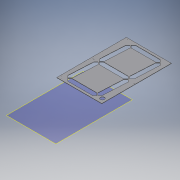
# Autodesk Inventor part: Cover_V2
Saved by Autodesk Inventor 2016 SP2 (Build 200236200, 236)
## iProperties
Created: 2018-06-10
Part Number: Cover_V2
Material: Generisch
Document SubType Name: Modeling
Designer: Nils
Density: 1 g/cm^3
Appearance: Vorgabe
Author: Nils
Autodesk Inventor part; units mm, degrees
ref_plane "YZ Plane" through (0, 0, 0) normal (1, 0, 0) x (0, 1, 0)
ref_plane "XZ Plane" through (0, 0, 0) normal (0, 1, 0) x (-1, 0, 0)
ref_plane "XY Plane" through (0, 0, 0) normal (0, 0, 1) x (1, 0, 0)
sketch "Skizze1" plane through (0, 0, 0) normal (0, 0, 1) x (1, 0, 0)
  line L0 (-29.0874, 239.038) -> (-29.0874, 85.837) projected
  line L1 (-29.0874, 85.837) -> (69.9128, 85.837) projected
  line L2 (-21.0874, 102.0037) -> (-18.2612, 155.9297) projected
  line L3 (-16.0874, 97.0037) -> (-21.0874, 102.0037) projected
  line L4 (-11.0874, 102.0037) -> (-16.0874, 97.0037) projected
  line L5 (-18.2612, 155.9297) -> (-13.2612, 160.9297) projected
  line L6 (-13.2612, 160.9297) -> (-8.2612, 155.9297) projected
  line L7 (44.0794, 90.837) -> (-9.9206, 90.837) projected
  line L8 (-9.9206, 90.837) -> (-14.9206, 95.837) projected
  line L9 (-14.9206, 95.837) -> (-9.9206, 100.837) projected
  line L10 (49.0794, 95.837) -> (44.0794, 90.837) projected
  line L11 (44.0794, 100.837) -> (49.0794, 95.837) projected
  line L12 (-9.9206, 100.837) -> (44.0794, 100.837)
  line L13 (-11.0874, 102.0037) -> (-8.2612, 155.9297)
  line L14 (-17.5791, 168.9453) -> (-14.753, 222.8713) projected
  line L15 (-12.5791, 163.9453) -> (-17.5791, 168.9453) projected
  line L16 (-7.5791, 168.9453) -> (-12.5791, 163.9453) projected
  line L17 (-14.753, 222.8713) -> (-9.753, 227.8713) projected
  line L18 (-9.753, 227.8713) -> (-4.753, 222.8713) projected
  line L19 (-3.5862, 224.038) -> (-8.5862, 229.038) projected
  line L20 (-8.5862, 229.038) -> (-3.5862, 234.038) projected
  line L21 (-3.5862, 234.038) -> (50.4138, 234.038) projected
  line L22 (50.4138, 234.038) -> (55.4138, 229.038) projected
  line L23 (55.4138, 229.038) -> (50.4138, 224.038) projected
  line L24 (51.5805, 222.8713) -> (56.5805, 227.8713) projected
  line L25 (56.5805, 227.8713) -> (61.5805, 222.8713) projected
  line L26 (61.5805, 222.8713) -> (58.7544, 168.9453) projected
  line L27 (58.7544, 168.9453) -> (53.7544, 163.9453) projected
  line L28 (53.7544, 163.9453) -> (48.7544, 168.9453) projected
  line L29 (-7.0945, 157.0964) -> (-12.0945, 162.0964) projected
  line L30 (-12.0945, 162.0964) -> (-7.0945, 167.0964) projected
  line L31 (-7.0945, 167.0964) -> (46.9055, 167.0964) projected
  line L32 (46.9055, 167.0964) -> (51.9055, 162.0964) projected
  line L33 (51.9055, 162.0964) -> (46.9055, 157.0964) projected
  line L34 (48.0722, 155.9297) -> (53.0722, 160.9297) projected
  line L35 (53.0722, 160.9297) -> (58.0722, 155.9297) projected
  line L36 (58.0722, 155.9297) -> (55.2461, 102.0037) projected
  line L37 (55.2461, 102.0037) -> (50.2461, 97.0037) projected
  line L38 (50.2461, 97.0037) -> (45.2461, 102.0037) projected
  line L39 (64.7975, 88.9856) -> (50.5282, 88.9856) construction
  line L40 (56.4128, 100.837) -> (66.9128, 100.837) construction
  line L41 (66.9128, 100.837) -> (66.9128, 90.837) construction
  line L42 (48.4128, 88.9856) -> (48.4128, 90.837) construction
  circle A0 centre (60.9128, 96.337) radius 4.5
  line L43 (45.2461, 102.0037) -> (48.0722, 155.9297)
  line L44 (46.9055, 157.0964) -> (-7.0945, 157.0964)
  line L45 (-7.5791, 168.9453) -> (-4.753, 222.8713)
  line L46 (-3.5862, 224.038) -> (50.4138, 224.038)
  line L47 (51.5805, 222.8713) -> (48.7544, 168.9453)
  line L48 (69.9128, 239.038) -> (-29.0874, 239.038) projected
  line L49 (69.9128, 85.837) -> (69.9128, 239.038) projected
  point P0 (0, 0)
  dimension "d2" = 9
  dimension "d3" = 4.5
  dimension "d4" = 4.5
  constraints: 14 end point, 4 point on line, 2 horizontal, 2 parallel, 1 centre point
  measures "d2" diameter of A0
  measures "d3" distance from line of L40 A0.centre
  measures "d4" horizontal distance of A0.centre L40.start
extrude "Extrusion2" add sketch "Skizze1" along normal blind 0.6
sketch "Skizze2" plane through (0, 0, 0) normal (0, 0, -1) x (-1, 0, 0)
  circle A0 centre (-64.9128, 162.0964) radius 2.4
  circle A1 centre (-64.9128, 234.038) radius 2.4
  circle A2 centre (24.0874, 234.038) radius 2.4
  circle A3 centre (24.0874, 162.0964) radius 2.4
  circle A4 centre (24.0874, 90.837) radius 2.4
  circle A5 centre (-64.9128, 105.837) radius 2.4
  circle A6 centre (-64.9128, 234.038) radius 2.5 projected
  circle A7 centre (24.0874, 234.038) radius 2.5 projected
  circle A8 centre (24.0874, 162.0964) radius 2.5 projected
  circle A9 centre (24.0874, 90.837) radius 2.5 projected
  circle A10 centre (-64.9128, 162.0964) radius 2.5 projected
  circle A11 centre (-64.9128, 105.837) radius 2.5 projected
  point P0 (0, 0)
  dimension "d7" = 4.8
  dimension "d8" = 4.8
  dimension "d9" = 4.8
  dimension "d10" = 4.8
  dimension "d11" = 4.8
  dimension "d14" = 4.8
  constraints: 6 centre point, 6 coincident
  measures "d7" diameter of A0
  measures "d8" diameter of A1
  measures "d9" diameter of A2
  measures "d10" diameter of A3
  measures "d11" diameter of A4
  measures "d14" diameter of A5
extrude "Extrusion3" add sketch "Skizze2" along normal blind 2.6 contours A0 | A1 | A2 | A3 | A4 | A5
ref_plane "Arbeitsebene1" through (20.4127, 47.5501, -21.1283) normal (0, 0, -1) x (-1, 0, 0)
equation "\"d4\" = d3"
equation "\"d8\" = d7"
equation "\"d9\" = d7"
equation "\"d10\" = d7"
equation "\"d11\" = d7"
equation "\"d14\" = d7"
